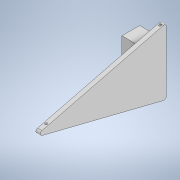
# Autodesk Inventor part: ت مهمه 3
Saved by Autodesk Inventor 2022 (Build 260153000, 153)
## iProperties
Created: 2021-07-14
Part Number: ت مهمه 3
Material: Generic
Document SubType Name: Sheet Metal
Designer: Nay
Density: 1 g/cm^3
Sheet Metal Rule: Default_mm
Appearance: Default
Author: Nay
Autodesk Inventor part; units mm, degrees
ref_plane "YZ Plane" through (0, 0, 0) normal (1, 0, 0) x (0, 1, 0)
ref_plane "XZ Plane" through (0, 0, 0) normal (0, 1, 0) x (-1, 0, 0)
ref_plane "XY Plane" through (0, 0, 0) normal (0, 0, 1) x (1, 0, 0)
sketch "Sketch1" plane through (0, 0, 0) normal (1, 0, 0) x (0, 1, 0)
  line L0 (7.5, 15) -> (-7.5, 15)
  line L1 (-7.5, 15) -> (-7.5, -15)
  line L2 (-7.5, -15) -> (7.5, -15)
  line L3 (7.5, -15) -> (7.5, 15)
  point P0 (0, 0)
  dimension "d0" = 30
  dimension "d1" = 15
  dimension "d2" = 7.5
  dimension "d3" = 15
  constraints: 8 end point, 2 parallel, 1 horizontal, 1 perpendicular
  measures "d0" distance of L2.end L0.start
  measures "d1" distance of L1.end L2.end
  measures "d2" distance from line of point (0, 0) L3
  measures "d3" distance from line of point (0, 0) L2
extrude "Extrusion1" add sketch "Sketch1" along normal blind 1
sketch "Sketch2" plane through (0, 7.5, 15) normal (0, 1, 0) x (1, 0, 0)
  circle A0 centre (0.5, 3.3701) radius 0.25
  circle A1 centre (0.5, 29.0879) radius 0.25
  line L0 (0, 30) -> (0, 0) projected
  point P0 (0, 15)
  dimension "d6" = 0.5
  dimension "d7" = 0.5
  dimension "d8" = 0.5
  dimension "d9" = 0.5
  constraints: 2 centre point
  measures "d6" diameter of A0
  measures "d7" diameter of A1
  measures "d8" distance from line of L0 A1.centre
  measures "d9" distance from line of L0 A0.centre
extrude "Extrusion2" cut sketch "Sketch2" against normal blind 20
sketch "Sketch3" plane through (1, 0, 0) normal (1, 0, 0) x (0, 0, -1)
  line L0 (15, 7.5) -> (-15, 0)
  line L1 (-15, 7.5) -> (-15, -7.5) projected
  line L2 (-15, -7.5) -> (15, -7.5) projected
  line L3 (15, -7.5) -> (-15, 0)
  point P0 (0, 0)
  constraints: 4 end point, 1 midpoint
extrude "Extrusion3" cut sketch "Sketch3" against normal blind 20
sketch "Sketch4" plane through (1, 0, 0) normal (1, 0, 0) x (0, 0, -1)
  line L0 (-15, 0) -> (15, -7.5) projected
  line L1 (15, 7.5) -> (-15, 0)
  line L2 (-15, 7.5) -> (-15, 0) projected
  line L3 (-15, 0) -> (-15, 7.5)
  line L4 (-15, 7.5) -> (15, 7.5)
  point P0 (0, 0)
  constraints: 6 end point, 1 collinear, 1 perpendicular
extrude "Extrusion4" cut sketch "Sketch4" against normal blind 20
fillet "Fillet1" radius 0.5 3 edges at (0.5, 0, 15) (0.5, 7.5, -15) (0.5, -7.5, -15)
sketch "Sketch5" plane through (0, 0, 0) normal (-1, 0, 0) x (0, 0, 1)
  line L0 (-15, -6.8596) -> (-15, 6.8596) projected
  line L1 (-15, -4) -> (-11, -4)
  line L2 (-11, -4) -> (-11, 4)
  line L3 (-11, 4) -> (-15, 4)
  line L4 (-15, 4) -> (-15, -4)
  line L5 (-14.5, -3.5) -> (-11.5, -3.5)
  line L6 (-11.5, -3.5) -> (-11.5, 3.5)
  line L7 (-11.5, 3.5) -> (-14.5, 3.5)
  line L8 (-14.5, 3.5) -> (-14.5, -3.5)
  point P0 (0, 0)
  dimension "d17" = 8
  dimension "d18" = 4
  dimension "d19" = 4
  dimension "d20" = 7
  dimension "d21" = 3
  dimension "d22" = 0.5
  dimension "d23" = 0.5
  constraints: 16 end point, 4 parallel, 2 horizontal, 2 perpendicular, 1 point on line
  measures "d17" distance of L1.end L2.end
  measures "d18" distance of L1.start L1.end
  measures "d19" distance from line of point (0, 0) L1
  measures "d20" distance of L7.end L5.start
  measures "d21" distance of L6.end L7.end
  measures "d22" distance between parallel lines of L2 L6
  measures "d23" distance between parallel lines of L1 L5
extrude "Extrusion5" add sketch "Sketch5" along normal blind 5 contours L0 L3 L2 L1 | L8 L7 L6 L5
sketch "Sketch6" plane through (-5, 0, 0) normal (-1, 0, 0) x (0, 0, 1)
  line L0 (-11.5, -3.5) -> (-14.5, -3.5)
  line L1 (-14.5, -3.5) -> (-14.5, 3.5)
  line L2 (-14.5, 3.5) -> (-11.5, 3.5)
  line L3 (-11.5, 3.5) -> (-11.5, -3.5)
  line L4 (-11, -4) -> (-11, 4) projected
  line L5 (-15, -4) -> (-11, -4) projected
  point P0 (0, 0)
  dimension "d26" = 7
  dimension "d27" = 3
  dimension "d28" = 0.5
  dimension "d29" = 0.5
  constraints: 8 end point, 2 parallel, 1 horizontal, 1 perpendicular
  measures "d26" distance of L0.end L1.end
  measures "d27" distance of L0.start L0.end
  measures "d28" distance between parallel lines of L4 L3
  measures "d29" distance between parallel lines of L5 L0
extrude "Extrusion6" cut sketch "Sketch6" against normal blind 5
equation "\"BendRadius\" = Thickness"
equation "\"BendReliefWidth\" = Thickness"
equation "\"BendReliefDepth\" = 0.5 * Thickness"
equation "\"CornerReliefSize\" = 4 * Thickness"
equation "\"MinimumRemnant\" = 2 * Thickness"
equation "\"TransitionRadius\" = BendRadius"
equation "\"JacobiRadiusSize\" = BendRadius"
equation "\"GapSize\" = Thickness"
equation "\"Thickness\" = 0.5"
body "Solid1"
